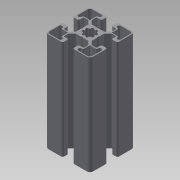
# Autodesk Inventor part: 45-4545-LITE
Saved by Autodesk Inventor 2013 (Build 170138000, 138)
## iProperties
Created: 2014-04-23
Part Number: 45-4545-LITE
Material: Generic
Document SubType Name: Modeling
Designer: Ross Bowman
Density: 1 g/cm^3
Engineer: Ross Bowman
Catalog Web Link: 8020.net
Vendor: 80/20 Inc.
Company: 80/20 Inc.
Author: Ross Bowman
Keywords: 80/20 , 8020 , T-Slot , Extrusion
Material: 6105-T5 Aluminum
Autodesk Inventor part; units mm, degrees
ref_plane "YZ Plane" through (0, 0, 0) normal (1, 0, 0) x (0, 1, 0)
ref_plane "XZ Plane" through (0, 0, 0) normal (0, 1, 0) x (-1, 0, 0)
ref_plane "XY Plane" through (0, 0, 0) normal (0, 0, 1) x (1, 0, 0)
sketch "Sketch1" plane through (0, 0, 0) normal (0, 0, 1) x (1, 0, 0)
  arc A0 (-0.7737, 4.9398) -> (-2.1534, 5.7864) centre (-1.7707, 4.8625) ccw
  arc A1 (0.7734, 4.9398) -> (-0.7737, 4.9398) centre (0, 0) ccw
  arc A2 (2.1531, 5.7865) -> (0.7734, 4.9398) centre (1.7705, 4.8626) ccw
  line L0 (2.1531, 5.7865) -> (2.5689, 5.6143)
  arc A3 (2.9458, 4.0401) -> (2.5689, 5.6143) centre (2.1862, 4.6904) ccw
  arc A4 (4.0399, 2.9461) -> (2.9458, 4.0401) centre (0, 0) ccw
  arc A5 (5.6142, 2.5692) -> (4.0399, 2.9461) centre (4.6903, 2.1865) ccw
  line L1 (5.6142, 2.5692) -> (5.7864, 2.1534)
  arc A6 (4.9398, 0.7737) -> (5.7864, 2.1534) centre (4.8625, 1.7707) ccw
  arc A7 (4.9398, -0.7734) -> (4.9398, 0.7737) centre (0, 0) ccw
  arc A8 (5.7865, -2.1531) -> (4.9398, -0.7734) centre (4.8626, -1.7705) ccw
  line L2 (5.7865, -2.1531) -> (5.6143, -2.5689)
  arc A9 (4.0401, -2.9458) -> (5.6143, -2.5689) centre (4.6904, -2.1862) ccw
  arc A10 (2.9461, -4.0399) -> (4.0401, -2.9458) centre (0, 0) ccw
  arc A11 (2.5692, -5.6142) -> (2.9461, -4.0399) centre (2.1865, -4.6903) ccw
  line L3 (2.5692, -5.6142) -> (2.1534, -5.7864)
  arc A12 (0.7737, -4.9398) -> (2.1534, -5.7864) centre (1.7707, -4.8625) ccw
  arc A13 (-0.7734, -4.9398) -> (0.7737, -4.9398) centre (0, 0) ccw
  arc A14 (-2.1531, -5.7865) -> (-0.7734, -4.9398) centre (-1.7705, -4.8626) ccw
  line L4 (-2.1531, -5.7865) -> (-2.5689, -5.6143)
  arc A15 (-2.9458, -4.0401) -> (-2.5689, -5.6143) centre (-2.1862, -4.6904) ccw
  arc A16 (-4.0399, -2.9461) -> (-2.9458, -4.0401) centre (0, 0) ccw
  arc A17 (-5.6142, -2.5692) -> (-4.0399, -2.9461) centre (-4.6903, -2.1865) ccw
  line L5 (-5.6142, -2.5692) -> (-5.7864, -2.1534)
  arc A18 (-4.9398, -0.7737) -> (-5.7864, -2.1534) centre (-4.8625, -1.7707) ccw
  arc A19 (-4.9398, 0.7734) -> (-4.9398, -0.7737) centre (0, 0) ccw
  arc A20 (-5.7865, 2.1531) -> (-4.9398, 0.7734) centre (-4.8626, 1.7705) ccw
  line L6 (-5.7865, 2.1531) -> (-5.6143, 2.5689)
  arc A21 (-4.0401, 2.9458) -> (-5.6143, 2.5689) centre (-4.6904, 2.1862) ccw
  arc A22 (-2.9461, 4.0399) -> (-4.0401, 2.9458) centre (0, 0) ccw
  arc A23 (-2.5692, 5.6142) -> (-2.9461, 4.0399) centre (-2.1865, 4.6903) ccw
  line L7 (-2.5692, 5.6142) -> (-2.1534, 5.7864)
  arc A24 (17.9765, 9.9875) -> (16.9765, 10.9875) centre (16.9765, 9.9875) ccw
  line L8 (16.9765, 10.9875) -> (11.4065, 10.9875)
  arc A25 (11.0265, 11.3675) -> (11.4065, 10.9875) centre (11.4065, 11.3675) ccw
  line L9 (11.0265, 11.3675) -> (11.0265, 16.9375)
  arc A26 (11.0265, 16.9375) -> (10.0265, 17.9375) centre (10.0265, 16.9375) ccw
  line L10 (10.0265, 17.9375) -> (9.5865, 17.9375)
  arc A27 (8.0865, 19.4375) -> (9.5865, 17.9375) centre (9.5865, 19.4375) ccw
  line L11 (8.0865, 19.4375) -> (8.0865, 19.9375)
  arc A28 (9.5865, 21.4375) -> (8.0865, 19.9375) centre (9.5865, 19.9375) ccw
  line L12 (9.5865, 21.4375) -> (19.1965, 21.4375)
  arc A29 (21.4765, 19.1575) -> (19.1965, 21.4375) centre (19.1965, 19.1575) ccw
  line L13 (21.4765, 19.1575) -> (21.4765, 9.5475)
  arc A30 (19.9765, 8.0475) -> (21.4765, 9.5475) centre (19.9765, 9.5475) ccw
  line L14 (19.9765, 8.0475) -> (19.4765, 8.0475)
  arc A31 (17.9765, 9.5475) -> (19.4765, 8.0475) centre (19.4765, 9.5475) ccw
  line L15 (17.9765, 9.5475) -> (17.9765, 9.9875)
  line L16 (6.2339, -7.9175) -> (0.9235, -7.9175)
  arc A32 (6.5026, -8.0288) -> (6.2339, -7.9175) centre (6.2339, -8.2975) ccw
  line L17 (9.9622, -11.4884) -> (6.5026, -8.0288)
  arc A33 (10.0735, -11.7571) -> (9.9622, -11.4884) centre (9.6935, -11.7571) ccw
  line L18 (10.0735, -16.0575) -> (10.0735, -11.7571)
  arc A34 (9.6935, -16.4375) -> (10.0735, -16.0575) centre (9.6935, -16.0575) ccw
  line L19 (6.6085, -16.4375) -> (9.6935, -16.4375)
  arc A35 (6.6085, -16.4375) -> (5.0885, -17.9575) centre (6.6085, -17.9575) ccw
  line L20 (5.0885, -20.9175) -> (5.0885, -17.9575)
  arc A36 (5.0885, -20.9175) -> (6.6085, -22.4375) centre (6.6085, -20.9175) ccw
  line L21 (19.5235, -22.4375) -> (6.6085, -22.4375)
  arc A37 (19.5235, -22.4375) -> (22.5235, -19.4375) centre (19.5235, -19.4375) ccw
  line L22 (22.5235, -6.5225) -> (22.5235, -19.4375)
  arc A38 (22.5235, -6.5225) -> (21.0035, -5.0025) centre (21.0035, -6.5225) ccw
  line L23 (18.0435, -5.0025) -> (21.0035, -5.0025)
  arc A39 (18.0435, -5.0025) -> (16.5235, -6.5225) centre (18.0435, -6.5225) ccw
  line L24 (16.5235, -9.6075) -> (16.5235, -6.5225)
  arc A40 (16.1435, -9.9875) -> (16.5235, -9.6075) centre (16.1435, -9.6075) ccw
  line L25 (11.8502, -9.9875) -> (16.1435, -9.9875)
  arc A41 (11.5815, -9.8762) -> (11.8502, -9.9875) centre (11.8502, -9.6075) ccw
  line L26 (8.1148, -6.4095) -> (11.5815, -9.8762)
  arc A42 (8.0035, -6.1408) -> (8.1148, -6.4095) centre (8.3835, -6.1408) ccw
  line L27 (8.0035, -0.8375) -> (8.0035, -6.1408)
  line L28 (7.4839, 0.0625) -> (8.0035, -0.8375)
  line L29 (8.0035, 0.9625) -> (7.4839, 0.0625)
  line L30 (8.0035, 6.2729) -> (8.0035, 0.9625)
  arc A43 (8.1148, 6.5416) -> (8.0035, 6.2729) centre (8.3835, 6.2729) ccw
  line L31 (11.5744, 10.0012) -> (8.1148, 6.5416)
  arc A44 (11.8431, 10.1125) -> (11.5744, 10.0012) centre (11.8431, 9.7325) ccw
  line L32 (16.1435, 10.1125) -> (11.8431, 10.1125)
  arc A45 (16.5235, 9.7325) -> (16.1435, 10.1125) centre (16.1435, 9.7325) ccw
  line L33 (16.5235, 6.6475) -> (16.5235, 9.7325)
  arc A46 (16.5235, 6.6475) -> (18.0435, 5.1275) centre (18.0435, 6.6475) ccw
  line L34 (21.0035, 5.1275) -> (18.0435, 5.1275)
  arc A47 (21.0035, 5.1275) -> (22.5235, 6.6475) centre (21.0035, 6.6475) ccw
  line L35 (22.5235, 19.5625) -> (22.5235, 6.6475)
  arc A48 (22.5235, 19.5625) -> (19.5235, 22.5625) centre (19.5235, 19.5625) ccw
  line L36 (6.6085, 22.5625) -> (19.5235, 22.5625)
  arc A49 (6.6085, 22.5625) -> (5.0885, 21.0425) centre (6.6085, 21.0425) ccw
  line L37 (5.0885, 18.0825) -> (5.0885, 21.0425)
  arc A50 (5.0885, 18.0825) -> (6.6085, 16.5625) centre (6.6085, 18.0825) ccw
  line L38 (9.6935, 16.5625) -> (6.6085, 16.5625)
  arc A51 (10.0735, 16.1825) -> (9.6935, 16.5625) centre (9.6935, 16.1825) ccw
  line L39 (10.0735, 11.8892) -> (10.0735, 16.1825)
  arc A52 (9.9622, 11.6205) -> (10.0735, 11.8892) centre (9.6935, 11.8892) ccw
  line L40 (6.4955, 8.1538) -> (9.9622, 11.6205)
  arc A53 (6.2268, 8.0425) -> (6.4955, 8.1538) centre (6.2268, 8.4225) ccw
  line L41 (0.9235, 8.0425) -> (6.2268, 8.0425)
  line L42 (0.0235, 7.5274) -> (0.9235, 8.0425)
  line L43 (-0.8765, 8.0425) -> (0.0235, 7.5274)
  line L44 (-6.1869, 8.0425) -> (-0.8765, 8.0425)
  arc A54 (-6.4556, 8.1538) -> (-6.1869, 8.0425) centre (-6.1869, 8.4225) ccw
  line L45 (-9.9152, 11.6134) -> (-6.4556, 8.1538)
  arc A55 (-10.0265, 11.8821) -> (-9.9152, 11.6134) centre (-9.6465, 11.8821) ccw
  line L46 (-10.0265, 16.1825) -> (-10.0265, 11.8821)
  arc A56 (-9.6465, 16.5625) -> (-10.0265, 16.1825) centre (-9.6465, 16.1825) ccw
  line L47 (-6.5615, 16.5625) -> (-9.6465, 16.5625)
  arc A57 (-6.5615, 16.5625) -> (-5.0415, 18.0825) centre (-6.5615, 18.0825) ccw
  line L48 (-5.0415, 21.0425) -> (-5.0415, 18.0825)
  arc A58 (-5.0415, 21.0425) -> (-6.5615, 22.5625) centre (-6.5615, 21.0425) ccw
  line L49 (-19.4765, 22.5625) -> (-6.5615, 22.5625)
  arc A59 (-19.4765, 22.5625) -> (-22.4765, 19.5625) centre (-19.4765, 19.5625) ccw
  line L50 (-22.4765, 6.6475) -> (-22.4765, 19.5625)
  arc A60 (-22.4765, 6.6475) -> (-20.9565, 5.1275) centre (-20.9565, 6.6475) ccw
  line L51 (-17.9965, 5.1275) -> (-20.9565, 5.1275)
  arc A61 (-17.9965, 5.1275) -> (-16.4765, 6.6475) centre (-17.9965, 6.6475) ccw
  line L52 (-16.4765, 9.7325) -> (-16.4765, 6.6475)
  arc A62 (-16.0965, 10.1125) -> (-16.4765, 9.7325) centre (-16.0965, 9.7325) ccw
  line L53 (-11.8032, 10.1125) -> (-16.0965, 10.1125)
  arc A63 (-11.5345, 10.0012) -> (-11.8032, 10.1125) centre (-11.8032, 9.7325) ccw
  line L54 (-8.0678, 6.5345) -> (-11.5345, 10.0012)
  arc A64 (-7.9565, 6.2658) -> (-8.0678, 6.5345) centre (-8.3365, 6.2658) ccw
  line L55 (-7.9565, 0.9625) -> (-7.9565, 6.2658)
  line L56 (-7.4369, 0.0625) -> (-7.9565, 0.9625)
  line L57 (-7.9565, -0.8375) -> (-7.4369, 0.0625)
  line L58 (-7.9565, -6.1479) -> (-7.9565, -0.8375)
  arc A65 (-8.0678, -6.4166) -> (-7.9565, -6.1479) centre (-8.3365, -6.1479) ccw
  line L59 (-11.5274, -9.8762) -> (-8.0678, -6.4166)
  arc A66 (-11.7961, -9.9875) -> (-11.5274, -9.8762) centre (-11.7961, -9.6075) ccw
  line L60 (-16.0965, -9.9875) -> (-11.7961, -9.9875)
  arc A67 (-16.4765, -9.6075) -> (-16.0965, -9.9875) centre (-16.0965, -9.6075) ccw
  line L61 (-16.4765, -6.5225) -> (-16.4765, -9.6075)
  arc A68 (-16.4765, -6.5225) -> (-17.9965, -5.0025) centre (-17.9965, -6.5225) ccw
  line L62 (-20.9565, -5.0025) -> (-17.9965, -5.0025)
  arc A69 (-20.9565, -5.0025) -> (-22.4765, -6.5225) centre (-20.9565, -6.5225) ccw
  line L63 (-22.4765, -19.4375) -> (-22.4765, -6.5225)
  arc A70 (-22.4765, -19.4375) -> (-19.4765, -22.4375) centre (-19.4765, -19.4375) ccw
  line L64 (-6.5615, -22.4375) -> (-19.4765, -22.4375)
  arc A71 (-6.5615, -22.4375) -> (-5.0415, -20.9175) centre (-6.5615, -20.9175) ccw
  line L65 (-5.0415, -17.9575) -> (-5.0415, -20.9175)
  arc A72 (-5.0415, -17.9575) -> (-6.5615, -16.4375) centre (-6.5615, -17.9575) ccw
  line L66 (-9.6465, -16.4375) -> (-6.5615, -16.4375)
  arc A73 (-10.0265, -16.0575) -> (-9.6465, -16.4375) centre (-9.6465, -16.0575) ccw
  line L67 (-10.0265, -11.7642) -> (-10.0265, -16.0575)
  arc A74 (-9.9152, -11.4955) -> (-10.0265, -11.7642) centre (-9.6465, -11.7642) ccw
  line L68 (-6.4485, -8.0288) -> (-9.9152, -11.4955)
  arc A75 (-6.1798, -7.9175) -> (-6.4485, -8.0288) centre (-6.1798, -8.2975) ccw
  line L69 (-0.8765, -7.9175) -> (-6.1798, -7.9175)
  line L70 (0.0235, -7.4024) -> (-0.8765, -7.9175)
  line L71 (0.9235, -7.9175) -> (0.0235, -7.4024)
  arc A76 (9.9875, -17.9765) -> (10.9875, -16.9765) centre (9.9875, -16.9765) ccw
  line L72 (10.9875, -16.9765) -> (10.9875, -11.4065)
  arc A77 (11.3675, -11.0265) -> (10.9875, -11.4065) centre (11.3675, -11.4065) ccw
  line L73 (11.3675, -11.0265) -> (16.9375, -11.0265)
  arc A78 (16.9375, -11.0265) -> (17.9375, -10.0265) centre (16.9375, -10.0265) ccw
  line L74 (17.9375, -10.0265) -> (17.9375, -9.5865)
  arc A79 (19.4375, -8.0865) -> (17.9375, -9.5865) centre (19.4375, -9.5865) ccw
  line L75 (19.4375, -8.0865) -> (19.9375, -8.0865)
  arc A80 (21.4375, -9.5865) -> (19.9375, -8.0865) centre (19.9375, -9.5865) ccw
  line L76 (21.4375, -9.5865) -> (21.4375, -19.1965)
  arc A81 (19.1575, -21.4765) -> (21.4375, -19.1965) centre (19.1575, -19.1965) ccw
  line L77 (19.1575, -21.4765) -> (9.5475, -21.4765)
  arc A82 (8.0475, -19.9765) -> (9.5475, -21.4765) centre (9.5475, -19.9765) ccw
  line L78 (8.0475, -19.9765) -> (8.0475, -19.4765)
  arc A83 (9.5475, -17.9765) -> (8.0475, -19.4765) centre (9.5475, -19.4765) ccw
  line L79 (9.5475, -17.9765) -> (9.9875, -17.9765)
  arc A84 (-9.9875, 17.9765) -> (-10.9875, 16.9765) centre (-9.9875, 16.9765) ccw
  line L80 (-10.9875, 16.9765) -> (-10.9875, 11.4065)
  arc A85 (-11.3675, 11.0265) -> (-10.9875, 11.4065) centre (-11.3675, 11.4065) ccw
  line L81 (-11.3675, 11.0265) -> (-16.9375, 11.0265)
  arc A86 (-16.9375, 11.0265) -> (-17.9375, 10.0265) centre (-16.9375, 10.0265) ccw
  line L82 (-17.9375, 10.0265) -> (-17.9375, 9.5865)
  arc A87 (-19.4375, 8.0865) -> (-17.9375, 9.5865) centre (-19.4375, 9.5865) ccw
  line L83 (-19.4375, 8.0865) -> (-19.9375, 8.0865)
  arc A88 (-21.4375, 9.5865) -> (-19.9375, 8.0865) centre (-19.9375, 9.5865) ccw
  line L84 (-21.4375, 9.5865) -> (-21.4375, 19.1965)
  arc A89 (-19.1575, 21.4765) -> (-21.4375, 19.1965) centre (-19.1575, 19.1965) ccw
  line L85 (-19.1575, 21.4765) -> (-9.5475, 21.4765)
  arc A90 (-8.0475, 19.9765) -> (-9.5475, 21.4765) centre (-9.5475, 19.9765) ccw
  line L86 (-8.0475, 19.9765) -> (-8.0475, 19.4765)
  arc A91 (-9.5475, 17.9765) -> (-8.0475, 19.4765) centre (-9.5475, 19.4765) ccw
  line L87 (-9.5475, 17.9765) -> (-9.9875, 17.9765)
  arc A92 (-17.9765, -9.9875) -> (-16.9765, -10.9875) centre (-16.9765, -9.9875) ccw
  line L88 (-16.9765, -10.9875) -> (-11.4065, -10.9875)
  arc A93 (-11.0265, -11.3675) -> (-11.4065, -10.9875) centre (-11.4065, -11.3675) ccw
  line L89 (-11.0265, -11.3675) -> (-11.0265, -16.9375)
  arc A94 (-11.0265, -16.9375) -> (-10.0265, -17.9375) centre (-10.0265, -16.9375) ccw
  line L90 (-10.0265, -17.9375) -> (-9.5865, -17.9375)
  arc A95 (-8.0865, -19.4375) -> (-9.5865, -17.9375) centre (-9.5865, -19.4375) ccw
  line L91 (-8.0865, -19.4375) -> (-8.0865, -19.9375)
  arc A96 (-9.5865, -21.4375) -> (-8.0865, -19.9375) centre (-9.5865, -19.9375) ccw
  line L92 (-9.5865, -21.4375) -> (-19.1965, -21.4375)
  arc A97 (-21.4765, -19.1575) -> (-19.1965, -21.4375) centre (-19.1965, -19.1575) ccw
  line L93 (-21.4765, -19.1575) -> (-21.4765, -9.5475)
  arc A98 (-19.9765, -8.0475) -> (-21.4765, -9.5475) centre (-19.9765, -9.5475) ccw
  line L94 (-19.9765, -8.0475) -> (-19.4765, -8.0475)
  arc A99 (-17.9765, -9.5475) -> (-19.4765, -8.0475) centre (-19.4765, -9.5475) ccw
  line L95 (-17.9765, -9.5475) -> (-17.9765, -9.9875)
  constraints: 200 point on circle, 192 end point, 100 centre point
extrude "Extrusion1" add sketch "Sketch1" against normal blind 100
body "Solid1"
